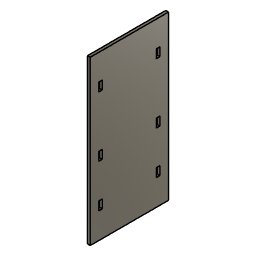
electricalPanel v3 (Autodesk Fusion 360 design; units mm, degrees)
Autodesk Fusion 360 part; units mm, degrees
sketch "Sketch1" plane through (0, 0, 0) normal (1, 0, 0) x (0, 1, 0)
  line L0 (0, 0) -> (45.6, 0)
  line L1 (45.6, 0) -> (45.6, 95)
  line L2 (45.6, 95) -> (0, 95)
  line L3 (0, 95) -> (0, 0)
  line L4 (5, 75) -> (7, 75)
  line L5 (7, 75) -> (7, 80)
  line L6 (7, 80) -> (5, 80)
  line L7 (5, 80) -> (5, 75)
  line L8 (38.6, 75) -> (40.6, 75)
  line L9 (40.6, 75) -> (40.6, 80)
  line L10 (40.6, 80) -> (38.6, 80)
  line L11 (38.6, 80) -> (38.6, 75)
  line L12 (5, 45) -> (7, 45)
  line L13 (7, 45) -> (7, 40)
  line L14 (7, 40) -> (5, 40)
  line L15 (5, 40) -> (5, 45)
  line L16 (38.6, 45) -> (40.6, 45)
  line L17 (40.6, 45) -> (40.6, 40)
  line L18 (40.6, 40) -> (38.6, 40)
  line L19 (38.6, 40) -> (38.6, 45)
  line L20 (5, 20) -> (7, 20)
  line L21 (7, 20) -> (7, 15)
  line L22 (7, 15) -> (5, 15)
  line L23 (5, 15) -> (5, 20)
  line L24 (38.6, 20) -> (40.6, 20)
  line L25 (40.6, 20) -> (40.6, 15)
  line L26 (40.6, 15) -> (38.6, 15)
  line L27 (38.6, 15) -> (38.6, 20)
  dimension "d1" = 45.6
  dimension "d2" = 95
  dimension "d3" = 2
  dimension "d4" = 2
  dimension "d5" = 5
  dimension "d6" = 5
  dimension "d7" = 5
  dimension "d8" = 15
  dimension "d9" = 30
  dimension "d10" = 15
  constraint horizontal L0
  constraint vertical L1
  constraint horizontal L2
  constraint vertical L3
  constraint coincident L0.start L3.end
  constraint horizontal L4
  constraint vertical L5
  constraint horizontal L6
  constraint vertical L7
  constraint horizontal L8
  constraint vertical L9
  constraint horizontal L10
  constraint vertical L11
  constraint horizontal L12
  constraint vertical L13
  constraint horizontal L14
  constraint vertical L15
  constraint horizontal L16
  constraint vertical L17
  constraint horizontal L18
  constraint vertical L19
  constraint horizontal L20
  constraint vertical L21
  constraint horizontal L22
  constraint vertical L23
  constraint horizontal L24
  constraint vertical L25
  constraint horizontal L26
  constraint vertical L27
  constraint vertical L13.end L20.end
  constraint vertical L5.end L12.end
  constraint vertical L10.end L16.start
  constraint vertical L18.end L24.start
  constraint vertical L17.end L24.end
  constraint vertical L9.end L16.end
  constraint vertical L6.end L12.start
  constraint vertical L14.end L20.start
  constraint horizontal L21.end L26.end
  constraint horizontal L20.end L24.start
  constraint horizontal L13.end L18.end
  constraint horizontal L12.end L16.start
  constraint horizontal L5.end L10.end
  constraint horizontal L4.end L8.start
  constraint equal L7 L15
  constraint equal L15 L23
  measures "d1" distance of L0.start L0.end
  measures "d2" distance of L0.start L2.end
  measures "d3" distance of L21.end L22.end
  measures "d4" distance of L25.end L26.end
  measures "d5" horizontal distance of L0.end L25.end
  measures "d6" horizontal distance of L0.start L22.end
  measures "d7" distance of L20.start L22.end
  measures "d8" vertical distance of L2.end L6.end
  measures "d9" distance of L4.start L12.start
  measures "d10" vertical distance of L0.start L22.end
extrude "Extrude1" add sketch "Sketch1" along normal blind 1.6
